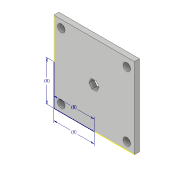
# Autodesk Inventor part: 103
Saved by Autodesk Inventor 2019 (Build 230136000, 136)
## iProperties
Created: 2019-11-17
Part Number: 103
Material: Generic
Document SubType Name: Modeling
Designer: Admin
Density: 1 g/cm^3
Appearance: Default
Author: Admin
Autodesk Inventor part; units mm, degrees
ref_plane "YZ Plane" through (0, 0, 0) normal (1, 0, 0) x (0, 1, 0)
ref_plane "XZ Plane" through (0, 0, 0) normal (0, 1, 0) x (-1, 0, 0)
ref_plane "XY Plane" through (0, 0, 0) normal (0, 0, 1) x (1, 0, 0)
sketch "Sketch1" plane through (0, 0, 0) normal (0, 0, 1) x (1, 0, 0)
  line L0 (0, 0) -> (160, 0)
  line L1 (160, 0) -> (160, 160)
  line L2 (160, 160) -> (0, 160)
  line L3 (0, 160) -> (0, 0)
  dimension "d0" = 160
  dimension "d1" = 160
  constraints: 8 end point, 2 parallel, 1 horizontal, 1 perpendicular
  measures "d0" distance of L2.end L1.end
  measures "d1" distance of L1.end L0.end
extrude "Extrusion1" add sketch "Sketch1" along normal blind 10
sketch "Sketch2" plane through (0, 0, 10) normal (0, 0, 1) x (1, 0, 0)
  line L0 (0, 0) -> (160, 0) projected
  line L1 (0, 0) -> (15, 0)
  line L2 (15, 0) -> (15, 15)
  line L3 (160, 160) -> (0, 160) projected
  line L4 (0, 160) -> (15, 160)
  line L5 (15, 160) -> (15, 145)
  line L6 (160, 0) -> (160, 160) projected
  line L7 (160, 160) -> (145, 160)
  line L8 (145, 160) -> (145, 143.5)
  line L9 (160, 0) -> (160, 15)
  line L10 (160, 15) -> (145, 15)
  circle A0 centre (15, 145) radius 7.5
  circle A1 centre (145, 143.5) radius 7.5
  circle A2 centre (145, 15) radius 7.5
  circle A3 centre (15, 15) radius 7.5
  dimension "d4" = 15
  dimension "d5" = 15
  dimension "d6" = 15
  dimension "d7" = 15
  dimension "d8" = 15
  dimension "d9" = 16.5
  dimension "d10" = 15
  dimension "d11" = 15
  dimension "d12" = 15
  dimension "d13" = 15
  dimension "d14" = 15
  dimension "d15" = 15
  constraints: 16 end point, 4 centre point, 4 coincident, 4 perpendicular, 4 point on line
  measures "d4" distance of L0.start L1.end
  measures "d5" distance of L1.end L2.end
  measures "d6" distance of L3.end L4.end
  measures "d7" distance of L4.end L5.end
  measures "d8" distance of L3.start L7.end
  measures "d9" distance of L7.end L8.end
  measures "d10" distance of L0.end L9.end
  measures "d11" distance of L9.end L10.end
  measures "d12" diameter of A0
  measures "d13" diameter of A1
  measures "d14" diameter of A2
  measures "d15" diameter of A3
extrude "Extrusion2" cut sketch "Sketch2" against normal blind 10
sketch "Sketch3" plane through (0, 0, 10) normal (0, 0, 1) x (1, 0, 0)
  line L0 (0, 160) -> (0, 0) projected
  line L1 (0, 0) -> (80, 0)
  line L2 (0, 0) -> (160, 0) projected
  line L3 (80, 0) -> (0, 0)
  line L4 (0, 0) -> (80, 0)
  dimension "d18" = 80
  dimension "d19" = 80
  dimension "d20" = 80
  constraints: 6 end point, 2 collinear, 1 midpoint
  measures "d18" distance of L0.end L1.end
  measures "d19" distance of L1.end L0.end
  measures "d20" distance of L0.end L1.end
sketch "Sketch4" plane through (0, 0, 10) normal (0, 0, 1) x (1, 0, 0)
  line L0 (0, 0) -> (160, 0) projected
  line L1 (0, 0) -> (0, 80)
  line L2 (0, 160) -> (0, 0) projected
  dimension "d21" = 80
  constraints: 2 end point, 1 midpoint
  measures "d21" distance of L0.start L1.end
sketch "Sketch5" plane through (0, 0, 10) normal (0, 0, 1) x (1, 0, 0)
  line L0 (0, 160) -> (0, 0) projected
  line L1 (0, 80) -> (80, 80)
  line L2 (84.0688, 89.1348) -> (89.9454, 81.0437)
  line L3 (89.9454, 81.0437) -> (85.8766, 71.9089)
  line L4 (85.8766, 71.9089) -> (75.9312, 70.8652)
  line L5 (75.9312, 70.8652) -> (70.0546, 78.9563)
  line L6 (70.0546, 78.9563) -> (74.1234, 88.0911)
  line L7 (74.1234, 88.0911) -> (84.0688, 89.1348)
  dimension "d22" = 80
  dimension "d23" = 10
  constraints: 14 end point, 1 coincident, 1 horizontal, 1 midpoint, 13 other
  measures "d22" distance of L1.start L1.end
  measures "d23" distance of L2.start L2.end
extrude "Extrusion3" cut sketch "Sketch5" against normal blind 10
body "Solid1"
